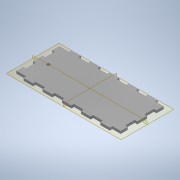
# Autodesk Inventor part: Plaat boven
Saved by Autodesk Inventor 2021 (Build 250183000, 183)
## iProperties
Created: 2021-01-09
Part Number: Plaat boven
Material: S235
Catalog Web Link: http://emmausbovenbouw.op-weg.be/
Vendor: Emmaüsinstituut Bovenbouw Aalter
Document SubType Name: Modeling
Designer: Antho
Engineer: Declercq St.
Manufacturer: Standard
Standards Organization: Custom
Density: 7.86 g/cm^3
Appearance: Steel
Manager: PJ / DCS
Company: Emmaüs Bovenbouw Aalter
Title: Algemene titel
Subject: Specifieke titel
Author: Antho
Keywords: Ruwe Ø xxxxx
Comments: Opmerking
Autodesk Inventor part; units mm, degrees
sketch "Sketch1" plane through (0, 0, 0) normal (0, 0, 1) x (1, 0, 0)
  line L0 (0, 2.8582) -> (0, -2.8582) construction
  line L1 (-5.7775, 0) -> (5.7775, 0) construction
  line L2 (-163, -75) -> (163, -75)
  line L3 (163, -75) -> (163, 75)
  line L4 (163, 75) -> (-163, 75)
  line L5 (-163, 75) -> (-163, -75)
  line L6 (-163, -75) -> (163, 75) construction
  line L7 (163, -75) -> (-163, 75) construction
  point P0 (0, 0)
  point P1 (0, 0)
  dimension "d0" = 326
  dimension "d1" = 150
  constraints: 16 end point, 4 midpoint, 2 horizontal, 2 parallel, 1 coincident, 1 perpendicular, 1 vertical
  measures "d0" distance of L4.end L3.end
  measures "d1" distance of L3.end L2.end
extrude "Extrusion1" add sketch "Sketch1" along normal blind 8
sketch "Sketch2" plane through (0, 0, 8) normal (0, 0, 1) x (1, 0, 0)
  line L0 (0, 0) -> (-130, 0)
  circle A0 centre (-130, 0) radius 5
  line L1 (-163, 75) -> (-163, -75) projected
  line L2 (-163, 0) -> (-163, 15)
  line L3 (-163, 15) -> (-163, -15)
  line L4 (-163, -15) -> (-163, -45)
  line L5 (-163, -45) -> (-163, -75)
  line L6 (-163, 15) -> (-163, 45)
  line L7 (-163, 45) -> (-163, 75)
  line L8 (-163, 15) -> (-155, 15)
  line L9 (-155, 15) -> (-155, 45)
  line L10 (-155, 45) -> (-163, 45)
  line L11 (-163, 45) -> (-163, 15)
  line L12 (-163, -15) -> (-155, -15)
  line L13 (-155, -15) -> (-155, -45)
  line L14 (-155, -45) -> (-163, -45)
  line L15 (-163, -45) -> (-163, -15)
  line L16 (-163, -75) -> (163, -75) projected
  line L17 (-163, -75) -> (-133, -75)
  line L18 (-133, -75) -> (-103, -75)
  line L19 (-103, -75) -> (-73, -75)
  line L20 (-73, -75) -> (-43, -75)
  line L21 (-43, -75) -> (-13, -75)
  line L22 (-13, -75) -> (17, -75)
  line L23 (17, -75) -> (47, -75)
  line L24 (47, -75) -> (77, -75)
  line L25 (77, -75) -> (107, -75)
  line L26 (107, -75) -> (137, -75)
  line L27 (137, -75) -> (167, -75)
  line L28 (-163, -75) -> (-133, -75)
  line L29 (-133, -75) -> (-133, -67)
  line L30 (-133, -67) -> (-163, -67)
  line L31 (-163, -67) -> (-163, -75)
  line L32 (-103, -75) -> (-73, -75)
  line L33 (-73, -75) -> (-73, -67)
  line L34 (-73, -67) -> (-103, -67)
  line L35 (-103, -67) -> (-103, -75)
  line L36 (-43, -75) -> (-13, -75)
  line L37 (-13, -75) -> (-13, -67)
  line L38 (-13, -67) -> (-43, -67)
  line L39 (-43, -67) -> (-43, -75)
  line L40 (17, -75) -> (47, -75)
  line L41 (47, -75) -> (47, -67)
  line L42 (47, -67) -> (17, -67)
  line L43 (17, -67) -> (17, -75)
  line L44 (77, -75) -> (107, -75)
  line L45 (107, -75) -> (107, -67)
  line L46 (107, -67) -> (77, -67)
  line L47 (77, -67) -> (77, -75)
  line L48 (137, -75) -> (163, -75)
  line L49 (163, -75) -> (163, -67)
  line L50 (163, -67) -> (137, -67)
  line L51 (137, -67) -> (137, -75)
  line L52 (163, 75) -> (-163, 75) projected
  line L53 (-163, 75) -> (-133, 75)
  line L54 (-133, 75) -> (-133, 67)
  line L55 (-133, 67) -> (-163, 67)
  line L56 (-163, 67) -> (-163, 75)
  line L57 (-103, 75) -> (-73, 75)
  line L58 (-73, 75) -> (-73, 67)
  line L59 (-73, 67) -> (-103, 67)
  line L60 (-103, 67) -> (-103, 75)
  line L61 (-43, 75) -> (-13, 75)
  line L62 (-13, 75) -> (-13, 67)
  line L63 (-13, 67) -> (-43, 67)
  line L64 (-43, 67) -> (-43, 75)
  line L65 (17, 75) -> (47, 75)
  line L66 (47, 75) -> (47, 67)
  line L67 (47, 67) -> (17, 67)
  line L68 (17, 67) -> (17, 75)
  line L69 (77, 75) -> (107, 75)
  line L70 (107, 75) -> (107, 67)
  line L71 (107, 67) -> (77, 67)
  line L72 (77, 67) -> (77, 75)
  line L73 (163, -75) -> (163, 75) projected
  line L74 (137, 75) -> (163, 75)
  line L75 (163, 75) -> (163, 67)
  line L76 (163, 67) -> (137, 67)
  line L77 (137, 67) -> (137, 75)
  line L78 (163, 0) -> (163, 15)
  line L79 (163, 15) -> (155, 15)
  line L80 (155, 15) -> (155, 45)
  line L81 (155, 45) -> (163, 45)
  line L82 (163, 45) -> (163, 15)
  line L83 (163, -15) -> (155, -15)
  line L84 (155, -15) -> (155, -45)
  line L85 (155, -45) -> (163, -45)
  line L86 (163, -45) -> (163, -15)
  dimension "d4" = 130
  dimension "d5" = 10
  dimension "d6" = 15
  dimension "d7" = 30
  dimension "d8" = 30
  dimension "d9" = 30
  dimension "d10" = 30
  dimension "d11" = 30
  dimension "d12" = 8
  dimension "d13" = 30
  dimension "d14" = 30
  dimension "d15" = 30
  dimension "d16" = 30
  dimension "d17" = 30
  dimension "d18" = 30
  dimension "d19" = 30
  dimension "d20" = 30
  dimension "d21" = 30
  dimension "d22" = 30
  dimension "d23" = 30
  dimension "d24" = 8
  dimension "d25" = 8
  dimension "d26" = 8
  constraints: 166 end point, 35 point on line, 32 parallel, 17 horizontal, 16 perpendicular, 2 collinear, 2 midpoint, 1 centre point, 1 coincident, 11 other
  measures "d4" distance of L0.start L0.end
  measures "d5" diameter of A0
  measures "d6" distance of L2.start L2.end
  measures "d7" distance of L2.end L3.end
  measures "d8" distance of L3.end L4.end
  measures "d9" distance of L4.end L1.end
  measures "d10" distance of L2.end L6.end
  measures "d11" distance of L6.end L1.start
  measures "d12" distance of L10.end L9.end
  measures "d13" distance of L1.end L17.end
  measures "d14" distance of L17.end L18.end
  measures "d15" distance of L18.end L19.end
  measures "d16" distance of L19.end L20.end
  measures "d17" distance of L20.end L21.end
  measures "d18" distance of L21.end L22.end
  measures "d19" distance of L22.end L23.end
  measures "d20" distance of L23.end L24.end
  measures "d21" distance of L24.end L25.end
  measures "d22" distance of L25.end L26.end
  measures "d23" distance of L26.end L27.end
  measures "d24" distance of L29.end L28.end
  measures "d25" distance of L53.end L54.end
  measures "d26" distance of L80.end L81.end
extrude "Extrusion2" cut sketch "Sketch2" against normal blind 8 contours A0 | L52 L54 L55 L1 | L10 L9 L8 L1 | L52 L58 L59 L60 | L52 L62 L63 L64 | L12 L13 L14 L1 | L52 L66 L67 L68 | L30 L29 L16 L1 | L52 L70 L71 L72 | L35 L34 L33 L16 | L52 L73 L76 L77 | L39 L38 L37 L16 | L73 L79 L80 L81 | L43 L42 L41 L16 | L47 L46 L45 L16 | L73 L85 L84 L83 | L51 L50 L49 L16
body "Solid1"
